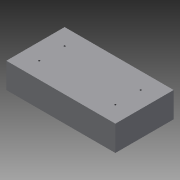
# Autodesk Inventor part: power supply
Saved by Autodesk Inventor 2013 (Build 170138000, 138)
## iProperties
Created: 2013-07-14
Part Number: power supply
Material: Generic
Document SubType Name: Modeling
Designer: employee
Density: 1 g/cm^3
Mass: 1236.07 g
Surface Area: 826.592 cm^2
Volume: 1236.07 cm^3
Author: employee
Autodesk Inventor part; units mm, degrees
ref_plane "YZ Plane" through (0, 0, 0) normal (1, 0, 0) x (0, 1, 0)
ref_plane "XZ Plane" through (0, 0, 0) normal (0, 1, 0) x (-1, 0, 0)
ref_plane "XY Plane" through (0, 0, 0) normal (0, 0, 1) x (1, 0, 0)
sketch "Sketch1" plane through (0, 0, 0) normal (0, 0, 1) x (1, 0, 0)
  line L0 (0, 0) -> (215, 0)
  line L1 (215, 0) -> (215, 115)
  line L2 (215, 115) -> (0, 115)
  line L3 (0, 115) -> (0, 0)
  dimension "d0" = 215
  dimension "d2" = 115
  constraints: 8 end point, 2 parallel, 1 coincident, 1 horizontal, 1 perpendicular
  measures "d0" distance of L0.start L0.end
  measures "d2" distance of L2.end L0.start
extrude "Extrusion1" add sketch "Sketch1" along normal blind 50
sketch "Sketch2" plane through (0, 0, 50) normal (0, 0, 1) x (1, 0, 0)
  line L0 (215, 0) -> (215, 115) projected
  line L1 (215, 115) -> (0, 115) projected
  line L2 (32.5, 82.5) -> (182.5, 82.5)
  line L3 (182.5, 82.5) -> (182.5, 32.5)
  line L4 (182.5, 32.5) -> (32.5, 32.5)
  line L5 (32.5, 32.5) -> (32.5, 82.5)
  point P0 (107.5, 82.5)
  point P1 (107.5, 115)
  point P2 (182.5, 57.5)
  point P3 (215, 57.5)
  dimension "d5" = 150
  dimension "d7" = 50
  constraints: 8 end point, 4 midpoint, 2 parallel, 1 horizontal, 1 horizontal alignment, 1 perpendicular, 1 vertical alignment
  measures "d5" distance of L3.end L4.end
  measures "d7" distance of L2.end L3.end
hole "Hole1" at (32.5, 82.5, 50) at (32.5, 32.5, 50) at (182.5, 32.5, 50) at (182.5, 82.5, 50) direction (0, 0, -1) diameter 3.242 depth 5 tip angle 118 thread size "M4x0.7" class "6H" standard "ANSI Metric M Profile"
body "Solid1"
